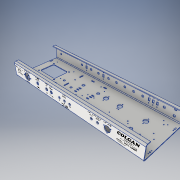
# Autodesk Inventor part: mainChassis
Saved by Autodesk Inventor 2018.3 (Build 223285000, 285)
## iProperties
Created: 2019-02-19
Part Number: mainChassis
Material: Aluminum 6061
Document SubType Name: Sheet Metal
Designer: RCCol
Density: 2.7 g/cm^3
Sheet Metal Rule: .125 thick aluminum
Appearance: Aluminum - Flat
Flat Pattern Width: 34.7497 cm
Flat Pattern Length: 60.325 cm
Flat Pattern Area: 2096.27 cm^2
Sheet Metal Width: 13.681 in
Sheet Metal Length: 23.750 in
Sheet Metal Area: 324.923 in^2
Author: RCCol
Autodesk Inventor part; units mm, degrees
ref_plane "YZ Plane" through (0, 0, 0) normal (1, 0, 0) x (0, 1, 0)
ref_plane "XZ Plane" through (0, 0, 0) normal (0, 1, 0) x (-1, 0, 0)
ref_plane "XY Plane" through (0, 0, 0) normal (0, 0, 1) x (1, 0, 0)
sketch "Sketch1" plane through (0, 0, 0) normal (0, 1, 0) x (-1, 0, 0)
  line L0 (0, 0) -> (-603.25, 0)
  line L1 (-603.25, 0) -> (-603.25, -204.47)
  line L2 (-603.25, -204.47) -> (0, -204.47)
  line L3 (0, -204.47) -> (0, 0)
  line L4 (0, 0) -> (-254, 0)
  line L5 (0, -79.375) -> (0, 0)
  dimension "d0" = 603.25
  dimension "d1" = 204.47
  constraints: 12 end point, 2 horizontal, 2 parallel, 1 perpendicular
  measures "d0" distance of L2.end L1.end
  measures "d1" distance of L1.end L0.end
extrude "Plate1" add sketch "Sketch1" along normal blind 3.175
sketch "Sketch2" plane through (0, 3.175, 0) normal (0, 1, 0) x (1, 0, 0)
  circle A0 centre (6.35, 38.735) radius 2.667
  line L0 (187.7208, 178.435) -> (187.6575, 164.4256)
  arc A1 (182.6575, 164.4256) -> (187.6575, 164.4256) centre (185.1575, 164.4256) ccw
  line L1 (182.6575, 164.4256) -> (182.6575, 178.435)
  arc A2 (187.7208, 178.435) -> (182.6575, 178.435) centre (185.1892, 178.5505) ccw
  line L2 (246.223, 175.935) -> (236.048, 175.935)
  arc A3 (236.048, 180.935) -> (236.048, 175.935) centre (236.048, 178.435) ccw
  line L3 (236.048, 180.935) -> (246.223, 180.935)
  arc A4 (246.223, 175.935) -> (246.223, 180.935) centre (245.9378, 178.435) ccw
  line L4 (308.1355, 110.435) -> (301.1355, 110.435)
  arc A5 (301.1355, 115.435) -> (301.1355, 110.435) centre (301.1355, 112.935) ccw
  line L5 (301.1355, 115.435) -> (308.1355, 115.435)
  arc A6 (308.1355, 110.435) -> (308.1355, 115.435) centre (308.1355, 112.935) ccw
  line L6 (308.1355, 99.735) -> (301.1355, 99.735)
  arc A7 (301.1355, 104.735) -> (301.1355, 99.735) centre (301.1355, 102.235) ccw
  line L7 (301.1355, 104.735) -> (308.1355, 104.735)
  arc A8 (308.1355, 99.735) -> (308.1355, 104.735) centre (308.1355, 102.235) ccw
  line L8 (243.048, 110.435) -> (236.048, 110.435)
  arc A9 (236.048, 115.435) -> (236.048, 110.435) centre (236.048, 112.935) ccw
  line L9 (236.048, 115.435) -> (243.048, 115.435)
  arc A10 (243.048, 110.435) -> (243.048, 115.435) centre (243.048, 112.935) ccw
  line L10 (243.048, 99.735) -> (236.048, 99.735)
  arc A11 (236.048, 104.735) -> (236.048, 99.735) centre (236.048, 102.235) ccw
  line L11 (236.048, 104.735) -> (243.048, 104.735)
  arc A12 (243.048, 99.735) -> (243.048, 104.735) centre (243.048, 102.235) ccw
  line L12 (305.694, 87.035) -> (298.694, 87.035)
  arc A13 (298.694, 92.035) -> (298.694, 87.035) centre (298.694, 89.535) ccw
  line L13 (298.694, 92.035) -> (305.694, 92.035)
  arc A14 (305.694, 87.035) -> (305.694, 92.035) centre (305.694, 89.535) ccw
  line L14 (239.251, 53.7042) -> (239.251, 57.4158)
  arc A15 (239.251, 57.4158) -> (238.6557, 58.0111) centre (238.6557, 57.4158) ccw
  line L15 (238.6557, 58.0111) -> (236.5443, 58.0111)
  arc A16 (236.5443, 58.0111) -> (235.949, 57.4158) centre (236.5443, 57.4158) ccw
  line L16 (235.949, 57.4158) -> (235.949, 53.7042)
  arc A17 (235.949, 53.7042) -> (236.5443, 53.1089) centre (236.5443, 53.7042) ccw
  line L17 (236.5443, 53.1089) -> (238.6557, 53.1089)
  arc A18 (238.6557, 53.1089) -> (239.251, 53.7042) centre (238.6557, 53.7042) ccw
  line L18 (239.251, 13.7042) -> (239.251, 17.4158)
  arc A19 (239.251, 17.4158) -> (238.6557, 18.0111) centre (238.6557, 17.4158) ccw
  line L19 (238.6557, 18.0111) -> (236.5443, 18.0111)
  arc A20 (236.5443, 18.0111) -> (235.949, 17.4158) centre (236.5443, 17.4158) ccw
  line L20 (235.949, 17.4158) -> (235.949, 13.7042)
  arc A21 (235.949, 13.7042) -> (236.5443, 13.1089) centre (236.5443, 13.7042) ccw
  line L21 (236.5443, 13.1089) -> (238.6557, 13.1089)
  arc A22 (238.6557, 13.1089) -> (239.251, 13.7042) centre (238.6557, 13.7042) ccw
  line L22 (175.751, 53.7042) -> (175.751, 57.4158)
  arc A23 (175.751, 57.4158) -> (175.1557, 58.0111) centre (175.1557, 57.4158) ccw
  line L23 (175.1557, 58.0111) -> (173.0443, 58.0111)
  arc A24 (173.0443, 58.0111) -> (172.449, 57.4158) centre (173.0443, 57.4158) ccw
  line L24 (172.449, 57.4158) -> (172.449, 53.7042)
  arc A25 (172.449, 53.7042) -> (173.0443, 53.1089) centre (173.0443, 53.7042) ccw
  line L25 (173.0443, 53.1089) -> (175.1557, 53.1089)
  arc A26 (175.1557, 53.1089) -> (175.751, 53.7042) centre (175.1557, 53.7042) ccw
  line L26 (175.751, 13.7042) -> (175.751, 17.4158)
  arc A27 (175.751, 17.4158) -> (175.1557, 18.0111) centre (175.1557, 17.4158) ccw
  line L27 (175.1557, 18.0111) -> (173.0443, 18.0111)
  arc A28 (173.0443, 18.0111) -> (172.449, 17.4158) centre (173.0443, 17.4158) ccw
  line L28 (172.449, 17.4158) -> (172.449, 13.7042)
  arc A29 (172.449, 13.7042) -> (173.0443, 13.1089) centre (173.0443, 13.7042) ccw
  line L29 (173.0443, 13.1089) -> (175.1557, 13.1089)
  arc A30 (175.1557, 13.1089) -> (175.751, 13.7042) centre (175.1557, 13.7042) ccw
  line L30 (112.251, 53.7042) -> (112.251, 57.4158)
  arc A31 (112.251, 57.4158) -> (111.6557, 58.0111) centre (111.6557, 57.4158) ccw
  line L31 (111.6557, 58.0111) -> (109.5443, 58.0111)
  arc A32 (109.5443, 58.0111) -> (108.949, 57.4158) centre (109.5443, 57.4158) ccw
  line L32 (108.949, 57.4158) -> (108.949, 53.7042)
  arc A33 (108.949, 53.7042) -> (109.5443, 53.1089) centre (109.5443, 53.7042) ccw
  line L33 (109.5443, 53.1089) -> (111.6557, 53.1089)
  arc A34 (111.6557, 53.1089) -> (112.251, 53.7042) centre (111.6557, 53.7042) ccw
  line L34 (112.251, 13.7042) -> (112.251, 17.4158)
  arc A35 (112.251, 17.4158) -> (111.6557, 18.0111) centre (111.6557, 17.4158) ccw
  line L35 (111.6557, 18.0111) -> (109.5443, 18.0111)
  arc A36 (109.5443, 18.0111) -> (108.949, 17.4158) centre (109.5443, 17.4158) ccw
  line L36 (108.949, 17.4158) -> (108.949, 13.7042)
  arc A37 (108.949, 13.7042) -> (109.5443, 13.1089) centre (109.5443, 13.7042) ccw
  line L37 (109.5443, 13.1089) -> (111.6557, 13.1089)
  arc A38 (111.6557, 13.1089) -> (112.251, 13.7042) centre (111.6557, 13.7042) ccw
  line L38 (48.751, 53.7042) -> (48.751, 57.4158)
  arc A39 (48.751, 57.4158) -> (48.1557, 58.0111) centre (48.1557, 57.4158) ccw
  line L39 (48.1557, 58.0111) -> (46.0443, 58.0111)
  arc A40 (46.0443, 58.0111) -> (45.449, 57.4158) centre (46.0443, 57.4158) ccw
  line L40 (45.449, 57.4158) -> (45.449, 53.7042)
  arc A41 (45.449, 53.7042) -> (46.0443, 53.1089) centre (46.0443, 53.7042) ccw
  line L41 (46.0443, 53.1089) -> (48.1557, 53.1089)
  arc A42 (48.1557, 53.1089) -> (48.751, 53.7042) centre (48.1557, 53.7042) ccw
  line L42 (48.751, 13.7042) -> (48.751, 17.4158)
  arc A43 (48.751, 17.4158) -> (48.1557, 18.0111) centre (48.1557, 17.4158) ccw
  line L43 (48.1557, 18.0111) -> (46.0443, 18.0111)
  arc A44 (46.0443, 18.0111) -> (45.449, 17.4158) centre (46.0443, 17.4158) ccw
  line L44 (45.449, 17.4158) -> (45.449, 13.7042)
  arc A45 (45.449, 13.7042) -> (46.0443, 13.1089) centre (46.0443, 13.7042) ccw
  line L45 (46.0443, 13.1089) -> (48.1557, 13.1089)
  arc A46 (48.1557, 13.1089) -> (48.751, 13.7042) centre (48.1557, 13.7042) ccw
  circle A47 centre (31.75, 177.5295) radius 1.5
  circle A48 centre (147.375, 75.2475) radius 1.65
  circle A49 centre (185.1575, 138.7475) radius 2.65
  circle A50 centre (259.135, 75.2475) radius 1.65
  circle A51 centre (536.2456, 75.5015) radius 1.65
  circle A52 centre (237.6, 35.56) radius 15.1
  circle A53 centre (174.1, 35.56) radius 15.1
  circle A54 centre (110.6, 35.56) radius 15.1
  circle A55 centre (47.1, 35.56) radius 15.1
  circle A56 centre (159.7575, 106.3403) radius 4.8
  circle A57 centre (212.2, 93.5148) radius 4.8
  circle A58 centre (309.5568, 135.335) radius 6.35
  circle A59 centre (234.6268, 135.335) radius 6.35
  circle A60 centre (269.35, 26.9408) radius 1.651
  circle A61 centre (511.2707, 37.4015) radius 9.525
  circle A62 centre (510.65, 51.6755) radius 1.651
  circle A63 centre (511.8914, 23.1275) radius 1.651
  circle A64 centre (514.7622, 134.3139) radius 9.525
  circle A65 centre (514.7622, 148.6014) radius 1.651
  circle A66 centre (514.7622, 120.0264) radius 1.651
  circle A67 centre (409.9872, 134.3139) radius 9.525
  circle A68 centre (409.9872, 148.6014) radius 1.651
  circle A69 centre (409.9872, 120.0264) radius 1.651
  circle A70 centre (348.0747, 134.3139) radius 9.525
  circle A71 centre (348.0747, 148.6014) radius 1.651
  circle A72 centre (348.0747, 120.0264) radius 1.651
  circle A73 centre (336.55, 37.1475) radius 9.525
  circle A74 centre (336.757, 22.8615) radius 1.651
  circle A75 centre (336.343, 51.4335) radius 1.651
  circle A76 centre (205.85, 26.9408) radius 1.651
  circle A77 centre (78.85, 26.9408) radius 1.651
  circle A78 centre (78.85, 63.0879) radius 1.651
  circle A79 centre (142.35, 26.035) radius 1.651
  circle A80 centre (193.85, 60.5908) radius 1.65
  circle A81 centre (217.85, 60.5908) radius 1.65
  circle A82 centre (205.85, 60.5908) radius 4.826
  circle A83 centre (137.16, 62.3578) radius 1.651
  circle A84 centre (548.7263, 68.2505) radius 4.826
  circle A85 centre (523.3263, 68.2505) radius 4.826
  circle A86 centre (474.4407, 24.0665) radius 2.3813
  circle A87 centre (501.8996, 75.999) radius 6.35
  circle A88 centre (474.4407, 95.504) radius 2.3813
  circle A89 centre (31.75, 159.385) radius 3.175
  circle A90 centre (127, 159.385) radius 3.175
  circle A91 centre (31.75, 83.185) radius 3.175
  circle A92 centre (127, 83.185) radius 3.175
  circle A93 centre (561.2206, 37.4015) radius 9.525
  circle A94 centre (561.1358, 51.6887) radius 1.651
  circle A95 centre (561.3053, 23.1143) radius 1.651
  circle A96 centre (78.85, 35.56) radius 3.2385
  circle A97 centre (142.35, 35.56) radius 3.2385
  circle A98 centre (205.85, 35.56) radius 3.2385
  circle A99 centre (269.35, 35.56) radius 3.2385
  circle A100 centre (6.35, 165.735) radius 2.667
  circle A101 centre (6.35, 158.3944) radius 1.5875
  circle A102 centre (6.35, 173.0756) radius 1.5875
  circle A103 centre (6.35, 31.3944) radius 1.5875
  circle A104 centre (6.35, 46.0756) radius 1.5875
  circle A105 centre (596.9, 38.735) radius 2.667
  circle A106 centre (596.9, 46.0756) radius 1.5875
  circle A107 centre (596.9, 31.3944) radius 1.5875
  circle A108 centre (596.9, 165.735) radius 2.667
  circle A109 centre (596.9, 173.0756) radius 1.5875
  circle A110 centre (596.9, 158.3944) radius 1.5875
  circle A111 centre (257.175, 61.9125) radius 3.2385
  circle A112 centre (298.0279, 22.861) radius 1.651
  circle A113 centre (298.195, 37.1475) radius 9.525
  circle A114 centre (298.3621, 51.434) radius 1.651
  circle A115 centre (431.8957, 46.0375) radius 14.9987
  circle A116 centre (431.8957, 68.8975) radius 1.651
  circle A117 centre (431.8957, 23.1775) radius 1.651
  arc A118 (43.053, 155.321) -> (35.179, 147.447) centre (43.053, 147.447) ccw
  line L46 (43.053, 155.321) -> (115.697, 155.321)
  arc A119 (123.571, 147.447) -> (115.697, 155.321) centre (115.697, 147.447) ccw
  line L47 (123.571, 147.447) -> (123.571, 95.123)
  arc A120 (115.697, 87.249) -> (123.571, 95.123) centre (115.697, 95.123) ccw
  line L48 (115.697, 87.249) -> (43.053, 87.249)
  arc A121 (35.179, 95.123) -> (43.053, 87.249) centre (43.053, 95.123) ccw
  line L49 (35.179, 95.123) -> (35.179, 147.447)
  line L50 (245.242, 87.035) -> (238.242, 87.035)
  arc A122 (238.242, 92.035) -> (238.242, 87.035) centre (238.242, 89.535) ccw
  line L51 (238.242, 92.035) -> (245.242, 92.035)
  arc A123 (245.242, 87.035) -> (245.242, 92.035) centre (245.242, 89.535) ccw
  line L52 (308.4045, 175.935) -> (298.2295, 175.935)
  arc A124 (298.2295, 180.935) -> (298.2295, 175.935) centre (298.2295, 178.435) ccw
  line L53 (298.2295, 180.935) -> (308.4045, 180.935)
  arc A125 (308.4045, 175.935) -> (308.4045, 180.935) centre (308.1193, 178.435) ccw
  line L54 (187.6575, 104.4569) -> (187.6575, 85.4475)
  arc A126 (182.6575, 85.4475) -> (187.6575, 85.4475) centre (185.1575, 85.4475) ccw
  line L55 (182.6575, 85.4475) -> (182.6415, 104.3746)
  arc A127 (187.6575, 104.4569) -> (182.6415, 104.3746) centre (185.1489, 104.4545) ccw
  circle A128 centre (316.1706, 160.7677) radius 1.8415
  circle A129 centre (316.1746, 106.5771) radius 1.8415
  circle A130 centre (416.475, 119.2676) radius 1.8415
  circle A131 centre (562.5222, 106.575) radius 1.8415
  circle A132 centre (562.5182, 160.7657) radius 1.8415
  circle A133 centre (552.2459, 176.288) radius 1.651
  circle A134 centre (571.2959, 168.5508) radius 1.651
  arc A135 (33.372, 18.6715) -> (19.656, 18.6715) centre (26.514, 12.8523) ccw
  arc A136 (19.656, 10.5435) -> (33.372, 10.5435) centre (26.514, 16.3626) ccw
  arc A137 (478.0682, 89.6801) -> (478.0692, 89.6801) centre (478.0687, 89.6801) ccw
  arc A138 (478.0692, 89.6801) -> (478.0682, 89.6801) centre (478.0687, 89.6801) ccw
  arc A139 (586.535, 89.6801) -> (586.536, 89.6801) centre (586.5355, 89.6801) ccw
  arc A140 (586.536, 89.6801) -> (586.535, 89.6801) centre (586.5355, 89.6801) ccw
  arc A141 (586.535, 89.6801) -> (586.536, 89.6801) centre (586.5355, 89.6801) ccw
  arc A142 (586.536, 89.6801) -> (586.535, 89.6801) centre (586.5355, 89.6801) ccw
  arc A143 (586.535, 14.4801) -> (586.536, 14.4801) centre (586.5355, 14.4801) ccw
  arc A144 (586.536, 14.4801) -> (586.535, 14.4801) centre (586.5355, 14.4801) ccw
  arc A145 (586.535, 14.4801) -> (586.536, 14.4801) centre (586.5355, 14.4801) ccw
  arc A146 (586.536, 14.4801) -> (586.535, 14.4801) centre (586.5355, 14.4801) ccw
  arc A147 (478.0682, 14.4801) -> (478.0692, 14.4801) centre (478.0687, 14.4801) ccw
  arc A148 (478.0692, 14.4801) -> (478.0682, 14.4801) centre (478.0687, 14.4801) ccw
  arc A149 (478.0682, 14.4801) -> (478.0692, 14.4801) centre (478.0687, 14.4801) ccw
  arc A150 (478.0692, 14.4801) -> (478.0682, 14.4801) centre (478.0687, 14.4801) ccw
  arc A151 (478.0682, 89.6801) -> (478.0692, 89.6801) centre (478.0687, 89.6801) ccw
  arc A152 (478.0692, 89.6801) -> (478.0682, 89.6801) centre (478.0687, 89.6801) ccw
  circle A153 centre (481.7263, 86.6923) radius 1.8415
  circle A154 centre (577.0271, 86.6923) radius 1.8415
  circle A155 centre (577.0271, 18.4679) radius 1.8415
  circle A156 centre (481.7263, 18.4679) radius 1.8415
  arc A157 (290.6947, 102.4493) -> (290.6957, 102.4493) centre (290.6952, 102.4493) ccw
  arc A158 (290.6957, 102.4493) -> (290.6947, 102.4493) centre (290.6952, 102.4493) ccw
  arc A159 (290.6947, 102.4493) -> (290.6957, 102.4493) centre (290.6952, 102.4493) ccw
  arc A160 (290.6957, 102.4493) -> (290.6947, 102.4493) centre (290.6952, 102.4493) ccw
  arc A161 (136.1947, 102.4493) -> (136.1957, 102.4493) centre (136.1952, 102.4493) ccw
  arc A162 (136.1957, 102.4493) -> (136.1947, 102.4493) centre (136.1952, 102.4493) ccw
  arc A163 (136.1947, 102.4493) -> (136.1957, 102.4493) centre (136.1952, 102.4493) ccw
  arc A164 (136.1957, 102.4493) -> (136.1947, 102.4493) centre (136.1952, 102.4493) ccw
  circle A165 centre (287.9348, 173.6201) radius 1.8415
  circle A166 centre (287.9348, 105.2941) radius 1.8415
  circle A167 centre (139.167, 173.6201) radius 1.8415
  circle A168 centre (139.167, 105.2941) radius 1.8415
  arc A169 (274.452, 90.8463) -> (274.453, 90.8463) centre (274.4525, 90.8463) ccw
  arc A170 (274.453, 90.8463) -> (274.452, 90.8463) centre (274.4525, 90.8463) ccw
  arc A171 (408.852, 90.8463) -> (408.853, 90.8463) centre (408.8525, 90.8463) ccw
  arc A172 (408.853, 90.8463) -> (408.852, 90.8463) centre (408.8525, 90.8463) ccw
  arc A173 (408.852, 90.8463) -> (408.853, 90.8463) centre (408.8525, 90.8463) ccw
  arc A174 (408.853, 90.8463) -> (408.852, 90.8463) centre (408.8525, 90.8463) ccw
  arc A175 (408.852, 14.2463) -> (408.853, 14.2463) centre (408.8525, 14.2463) ccw
  arc A176 (408.853, 14.2463) -> (408.852, 14.2463) centre (408.8525, 14.2463) ccw
  arc A177 (408.852, 14.2463) -> (408.853, 14.2463) centre (408.8525, 14.2463) ccw
  arc A178 (408.853, 14.2463) -> (408.852, 14.2463) centre (408.8525, 14.2463) ccw
  arc A179 (274.452, 14.2463) -> (274.453, 14.2463) centre (274.4525, 14.2463) ccw
  arc A180 (274.453, 14.2463) -> (274.452, 14.2463) centre (274.4525, 14.2463) ccw
  arc A181 (274.452, 14.2463) -> (274.453, 14.2463) centre (274.4525, 14.2463) ccw
  arc A182 (274.453, 14.2463) -> (274.452, 14.2463) centre (274.4525, 14.2463) ccw
  arc A183 (274.452, 90.8463) -> (274.453, 90.8463) centre (274.4525, 90.8463) ccw
  arc A184 (274.453, 90.8463) -> (274.452, 90.8463) centre (274.4525, 90.8463) ccw
  circle A185 centre (278.2879, 87.3221) radius 1.8415
  circle A186 centre (278.2879, 17.8785) radius 1.8415
  circle A187 centre (405.4149, 17.8785) radius 1.8415
  circle A188 centre (405.4149, 87.3221) radius 1.8415
  line L56 (19.656, 18.6715) -> (19.656, 10.5435)
  line L57 (33.372, 18.6715) -> (33.372, 10.5435)
  dimension "GapSize" = 3.175
  constraints: 196 point on circle, 189 centre point, 116 end point
sketch "Sketch3" plane through (603.25, 0, -3.175) normal (0, 0, 1) x (1, 0, 0)
  line L0 (-603.25, 0) -> (0, 0)
  line L1 (0, 0) -> (0, 63.5)
  line L2 (0, 63.5) -> (-603.25, 63.5)
  line L3 (-603.25, 63.5) -> (-603.25, 0)
  constraints: 6 end point, 1 horizontal, 1 perpendicular, 1 vertical
edge flange "Flange1" height 63.5 angle 90 thickness 3.175 bend radius 3.175 thickness toward (0, 0, 1) relief straight relief width 3.175 relief depth 1.5875 edges at (301.625, 3.175, 0) wall of the first edge with corners at (0, 0, -3.175) (603.25, 0, -3.175) (603.25, 63.5, -3.175) (0, 63.5, -3.175)
bend "Bend1"
corner "Corner1"
sketch "Sketch4" plane through (603.25, 60.325, 0) normal (0, 1, 0) x (-1, 0, 0)
  line L0 (603.25, 0) -> (0, 0)
  line L1 (0, 0) -> (0, -19.05)
  line L2 (0, -19.05) -> (603.25, -19.05)
  line L3 (603.25, -19.05) -> (603.25, 0)
  constraints: 6 end point, 1 horizontal, 1 perpendicular, 1 vertical
edge flange "Flange2" height 19.05 angle 90 thickness 3.175 bend radius 3.175 thickness toward (0, 1, 0) relief straight relief width 3.175 relief depth 1.5875 edges at (301.625, 63.5, -3.175) wall of the first edge with corners at (0, 60.325, 0) (603.25, 60.325, 0) (603.25, 60.325, -19.05) (0, 60.325, -19.05)
bend "Bend2"
corner "Corner2"
sketch "Sketch5" plane through (0, 6.35, 0) normal (0, 0, 1) x (1, 0, 0)
  circle A0 centre (99.805, 25.4) radius 1.778
  circle A1 centre (57.895, 25.4) radius 1.778
  line L0 (148.065, 22.0907) -> (148.065, 28.7093)
  line L1 (136.635, 22.0907) -> (136.635, 28.7093)
  arc A2 (136.635, 22.0907) -> (148.065, 22.0907) centre (142.35, 25.4) ccw
  arc A3 (148.065, 28.7093) -> (136.635, 28.7093) centre (142.35, 25.4) ccw
  line L2 (193.9018, 20.2386) -> (192.3982, 20.2386)
  arc A4 (193.9018, 19.2226) -> (192.3982, 19.2226) centre (193.15, 25.4) ccw
  line L3 (192.3982, 20.2386) -> (192.3982, 19.2226)
  line L4 (193.9018, 19.2226) -> (193.9018, 20.2386)
  line L5 (219.3018, 20.2386) -> (217.7982, 20.2386)
  arc A5 (219.3018, 19.2226) -> (217.7982, 19.2226) centre (218.55, 25.4) ccw
  line L6 (217.7982, 20.2386) -> (217.7982, 19.2226)
  line L7 (219.3018, 19.2226) -> (219.3018, 20.2386)
  circle A6 centre (261.3213, 25.4) radius 4.7625
  circle A7 centre (286.7213, 25.4) radius 4.7625
  circle A8 centre (312.1213, 25.4) radius 4.7625
  circle A9 centre (409.575, 25.5399) radius 4.7625
  circle A10 centre (434.975, 25.5399) radius 4.7625
  circle A11 centre (473.075, 25.5399) radius 12.1031
  circle A12 centre (460.2734, 32.9821) radius 1.778
  circle A13 centre (485.8766, 32.9821) radius 1.778
  circle A14 centre (473.075, 10.7317) radius 1.778
  line L8 (136.635, 28.7093) -> (148.065, 28.7093)
  line L9 (148.065, 28.7093) -> (148.065, 22.0907)
  line L10 (148.065, 22.0907) -> (136.635, 22.0907)
  line L11 (136.635, 22.0907) -> (136.635, 28.7093)
  arc A15 (148.065, 28.7093) -> (136.635, 28.7093) centre (142.35, 25.4) ccw
  arc A16 (136.635, 22.0907) -> (148.065, 22.0907) centre (142.35, 25.4) ccw
  arc A17 (136.635, 22.0907) -> (148.065, 22.0907) centre (142.35, 25.4) ccw
  arc A18 (193.9018, 19.2226) -> (192.3982, 19.2226) centre (193.15, 25.4) ccw
  line L12 (193.9018, 19.2226) -> (193.9018, 20.2386)
  line L13 (192.3982, 20.2386) -> (192.3982, 19.2226)
  circle A19 centre (78.85, 25.4) radius 15.875
  line L14 (193.9018, 26.5886) -> (192.3982, 26.5886)
  line L15 (192.3982, 26.5886) -> (192.3982, 25.5726)
  line L16 (193.9018, 25.5726) -> (193.9018, 26.5886)
  line L17 (219.3018, 26.5886) -> (217.7982, 26.5886)
  line L18 (217.7982, 26.5886) -> (217.7982, 25.5726)
  line L19 (219.3018, 25.5726) -> (219.3018, 26.5886)
  point P0 (0, -6.35)
  dimension "GapSize" = 3.175
  constraints: 40 end point, 23 point on circle, 20 centre point, 5 point on line, 2 parallel, 1 concentric, 1 horizontal, 1 perpendicular, 1 vertical
extrude "Cut2" cut sketch "Sketch5" against normal blind 3.175
sketch "Sketch6" plane through (0, 0, -201.295) normal (0, 0, -1) x (-1, 0, 0)
  line L0 (-603.25, 0) -> (0, 0)
  line L1 (0, 0) -> (0, 63.5)
  line L2 (0, 63.5) -> (-603.25, 63.5)
  line L3 (-603.25, 63.5) -> (-603.25, 0)
  constraints: 6 end point, 1 horizontal, 1 perpendicular, 1 vertical
edge flange "Flange3" height 63.5 angle 90 thickness 3.175 bend radius 3.175 thickness toward (0, 0, -1) relief straight relief width 3.175 relief depth 1.5875 edges at (301.625, 3.175, -204.47) wall of the first edge with corners at (603.25, 0, -201.295) (0, 0, -201.295) (0, 63.5, -201.295) (603.25, 63.5, -201.295)
bend "Bend3"
corner "Corner3"
sketch "Sketch7" plane through (0, 60.325, -204.47) normal (0, 1, 0) x (-1, 0, 0)
  line L0 (-603.25, 0) -> (0, 0)
  line L1 (0, 0) -> (0, 19.05)
  line L2 (0, 19.05) -> (-603.25, 19.05)
  line L3 (-603.25, 19.05) -> (-603.25, 0)
  constraints: 6 end point, 1 horizontal, 1 perpendicular, 1 vertical
edge flange "Flange4" height 19.05 angle 90 thickness 3.175 bend radius 3.175 thickness toward (0, 1, 0) relief straight relief width 3.175 relief depth 1.5875 edges at (301.625, 63.5, -201.295) wall of the first edge with corners at (603.25, 60.325, -204.47) (0, 60.325, -204.47) (0, 60.325, -185.42) (603.25, 60.325, -185.42)
bend "Bend4"
corner "Corner4"
sketch "Sketch8" plane through (603.25, 6.35, -204.47) normal (0, 0, -1) x (-1, 0, 0)
  line L0 (0, -6.35) -> (603.25, -6.35)
  line L1 (603.25, -6.35) -> (603.25, 57.15)
  line L2 (603.25, 57.15) -> (0, 57.15)
  line L3 (0, 57.15) -> (0, -6.35)
  circle A0 centre (31.9541, 38.1) radius 4.7625
  circle A1 centre (70.0541, 25.4) radius 4.7625
  circle A2 centre (190.9581, 25.4) radius 4.7625
  circle A3 centre (305.2581, 25.4) radius 4.7625
  circle A4 centre (444.9581, 25.4) radius 4.7625
  circle A5 centre (394.1581, 25.4) radius 4.7625
  circle A6 centre (356.0581, 25.4) radius 4.7625
  circle A7 centre (267.1581, 25.4) radius 4.7625
  circle A8 centre (229.0581, 25.4) radius 4.7625
  circle A9 centre (152.8581, 25.4) radius 4.7625
  circle A10 centre (31.9541, 12.7) radius 4.7625
  circle A11 centre (31.9541, 12.7) radius 4.7625
  circle A12 centre (152.8581, 25.4) radius 4.7625
  circle A13 centre (229.0581, 25.4) radius 4.7625
  circle A14 centre (267.1581, 25.4) radius 4.7625
  circle A15 centre (356.0581, 25.4) radius 4.7625
  circle A16 centre (394.1581, 25.4) radius 4.7625
  circle A17 centre (444.9581, 25.4) radius 4.7625
  circle A18 centre (305.2581, 25.4) radius 4.7625
  circle A19 centre (190.9581, 25.4) radius 4.7625
  circle A20 centre (70.0541, 25.4) radius 4.7625
  circle A21 centre (31.9541, 38.1) radius 4.7625
  circle A22 centre (571.5, 25.4) radius 3.9624
  circle A23 centre (95.4541, 39.6875) radius 1.7272
  circle A24 centre (95.4541, 11.1125) radius 1.7272
  circle A25 centre (111.4561, 39.6875) radius 1.7272
  circle A26 centre (111.4561, 11.1125) radius 1.7272
  circle A27 centre (127.4581, 39.6875) radius 1.7272
  circle A28 centre (127.4581, 11.1125) radius 1.7272
  circle A29 centre (330.6581, 39.6875) radius 1.7272
  circle A30 centre (330.6581, 11.1125) radius 1.7272
  circle A31 centre (419.5581, 39.6875) radius 1.7272
  circle A32 centre (419.5581, 11.1125) radius 1.7272
  line L4 (130.8871, 31.496) -> (130.8871, 19.304)
  line L5 (130.8871, 19.304) -> (124.0291, 19.304)
  line L6 (124.0291, 19.304) -> (124.0291, 31.496)
  line L7 (124.0291, 31.496) -> (130.8871, 31.496)
  line L8 (114.8851, 31.496) -> (114.8851, 19.304)
  line L9 (114.8851, 19.304) -> (108.0271, 19.304)
  line L10 (108.0271, 19.304) -> (108.0271, 31.496)
  line L11 (108.0271, 31.496) -> (114.8851, 31.496)
  line L12 (98.8831, 31.496) -> (98.8831, 19.304)
  line L13 (98.8831, 19.304) -> (92.0251, 19.304)
  line L14 (92.0251, 19.304) -> (92.0251, 31.496)
  line L15 (92.0251, 31.496) -> (98.8831, 31.496)
  line L16 (334.0871, 31.496) -> (334.0871, 19.304)
  line L17 (334.0871, 19.304) -> (327.2291, 19.304)
  line L18 (327.2291, 19.304) -> (327.2291, 31.496)
  line L19 (327.2291, 31.496) -> (334.0871, 31.496)
  line L20 (422.9871, 31.496) -> (422.9871, 19.304)
  line L21 (422.9871, 19.304) -> (416.1291, 19.304)
  line L22 (416.1291, 19.304) -> (416.1291, 31.496)
  line L23 (416.1291, 31.496) -> (422.9871, 31.496)
  dimension "GapSize" = 3.175
  constraints: 48 end point, 33 centre point
extrude "Cut3" cut sketch "Sketch8" against normal blind 3.175 contours A0 | A1 | A2 | A3 | A4 | A5 | A6 | A7 | A8 | A9 | A10 | A22 | A23 | A24 | A25 | A26 | A27 | A28 | A29 | A30 | A31 | A32 | L4 L5 L6 L7 | L8 L9 L10 L11 | L12 L13 L14 L15 | L16 L17 L18 L19 | L20 L21 L22 L23
sketch "Sketch9" plane through (603.25, 6.35, -204.47) normal (0, 0, -1) x (-1, 0, 0)
  line L0 (0, 50.8) -> (0, 53.975) projected
  line L1 (0, 53.975) -> (603.25, 53.975) projected
  line L2 (603.25, 53.975) -> (0, 53.975) projected
  line L3 (0, 50.8) -> (0, 0) projected
  line L4 (0, 50.8) -> (0, 0) projected
  line L5 (0, 50.8) -> (603.2512, 50.8) construction
  line L6 (603.2512, 50.8) -> (603.2512, -0.0001) construction
  line L7 (603.2512, -0.0001) -> (0, -0.0001) construction
  line L8 (0, -0.0001) -> (0, 50.8) construction
  point P0 (603.25, -6.35)
  constraints: 2 other
decal "Decal1"
sketch "Sketch10" plane through (0, 6.35, 0) normal (0, 0, 1) x (1, 0, 0)
  line L0 (0, 53.975) -> (0, 50.8) projected
  line L1 (0, 53.975) -> (603.2512, 53.975) construction
  line L2 (603.2512, 53.975) -> (603.2512, -3.1751) construction
  line L3 (603.2512, -3.1751) -> (0, -3.1751) construction
  line L4 (0, -3.1751) -> (0, 53.975) construction
  point P0 (0, -6.35)
  constraints: 2 other
decal "Decal2"
sketch "Sketch11" plane through (0, 3.175, 0) normal (0, 1, 0) x (1, 0, 0)
  line L0 (327.7837, 182.0084) -> (581.4999, 182.0084) construction
  line L1 (581.4999, 182.0084) -> (581.4999, 102.7644) construction
  line L2 (581.4999, 102.7644) -> (327.7837, 102.7644) construction
  line L3 (327.7837, 102.7644) -> (327.7837, 182.0084) construction
  line L4 (137.2091, 179.1073) -> (295.4903, 179.1073) construction
  line L5 (295.4903, 179.1073) -> (295.4903, 100.0089) construction
  line L6 (295.4903, 100.0089) -> (137.2091, 100.0089) construction
  line L7 (137.2091, 100.0089) -> (137.2091, 179.1073) construction
  line L8 (481.5672, 92.8982) -> (586.4692, 92.8982) construction
  line L9 (586.4692, 92.8982) -> (586.4692, 13.4373) construction
  line L10 (586.4692, 13.4373) -> (481.5672, 13.4373) construction
  line L11 (481.5672, 13.4373) -> (481.5672, 92.8982) construction
  point P0 (0, 0)
  constraints: 6 other
extrude "Cut4" cut sketch "Sketch2" against normal blind 3.175 contours A0 | L0 A1 L1 A2 | L2 A3 L3 A4 | L4 A5 L5 A6 | L6 A7 L7 A8 | L8 A9 L9 A10 | L10 A11 L11 A12 | L12 A13 L13 A14 | A18 L17 A17 L16 A16 L15 A15 L14 | A22 L21 A21 L20 A20 L19 A19 L18 | A26 L25 A25 L24 A24 L23 A23 L22 | A30 L29 A29 L28 A28 L27 A27 L26 | A34 L33 A33 L32 A32 L31 A31 L30 | A38 L37 A37 L36 A36 L35 A35 L34 | A42 L41 A41 L40 A40 L39 A39 L38 | A46 L45 A45 L44 A44 L43 A43 L42 | A47 | A48 | A49 | A50 | A51 | A52 | A53 | A54 | A55 | A56 | A57 | A58 | A59 | A60 | A61 | A62 | A63 | A64 | A65 | A66 | A67 | A68 | A69 | A70 | A71 | A72 | A73 | A74 | A75 | A76 | A77 | A78 | A79 | A80 | A81 | A82 | A83 | A84 | A85 | A86 | A87 | A88 | A89 | A90 | A91 | A92 | A93 | A94 | A95 | A96 | A97 | A98 | A99 | A100 | A101 | A102 | A103 | A104 | A105 | A106 | A107 | A108 | A109 | A110 | A111 | A112 | A113 | A114 | A115 | A116 | A117 | L46 A119 L47 A120 L48 A121 L49 A118 | L50 A122 L51 A123 | L52 A124 L53 A125 | L54 A126 L55 A127 | A128 | A129 | A130 | A131 | A132 | A133 | A134 | L57 A136 L56 A135 | A153 | A154 | A155 | A156 | A165 | A166 | A167 | A168 | A185 | A186 | A187 | A188
equation "\"GapSize\" = Thickness"
equation "\"d27\" = Thickness"
equation "\"d49\" = Thickness"
equation "\"d2\" = Thickness"
equation "\"d5\" = BendReliefWidth"
equation "\"d6\" = BendReliefDepth"
equation "\"d7\" = MinimumRemnant"
equation "\"d8\" = TransitionRadius"
equation "\"d11\" = BendRadius"
equation "\"d12\" = CornerReliefSize"
equation "\"d13\" = GapSize"
equation "\"d14\" = JacobiRadiusSize"
equation "\"d17\" = BendReliefWidth"
equation "\"d18\" = BendReliefDepth"
equation "\"d19\" = MinimumRemnant"
equation "\"d20\" = TransitionRadius"
equation "\"d23\" = BendRadius"
equation "\"d24\" = CornerReliefSize"
equation "\"d25\" = GapSize"
equation "\"d26\" = JacobiRadiusSize"
equation "\"d29\" = BendReliefWidth"
equation "\"d30\" = BendReliefDepth"
equation "\"d31\" = MinimumRemnant"
equation "\"d32\" = TransitionRadius"
equation "\"d35\" = BendRadius"
equation "\"d36\" = CornerReliefSize"
equation "\"d37\" = GapSize"
equation "\"d38\" = JacobiRadiusSize"
equation "\"d39\" = BendReliefWidth"
equation "\"d40\" = BendReliefDepth"
equation "\"d41\" = MinimumRemnant"
equation "\"d42\" = TransitionRadius"
equation "\"d45\" = BendRadius"
equation "\"d46\" = CornerReliefSize"
equation "\"d47\" = GapSize"
equation "\"d48\" = JacobiRadiusSize"
equation "\"BendRadius\" = Thickness"
equation "\"BendReliefWidth\" = Thickness"
equation "\"BendReliefDepth\" = 0.5 * Thickness"
equation "\"CornerReliefSize\" = 4 * Thickness"
equation "\"MinimumRemnant\" = 2 * Thickness"
equation "\"TransitionRadius\" = BendRadius"
equation "\"JacobiRadiusSize\" = BendRadius"
equation "\"Thickness\" = 3.175"
body "Solid1"
